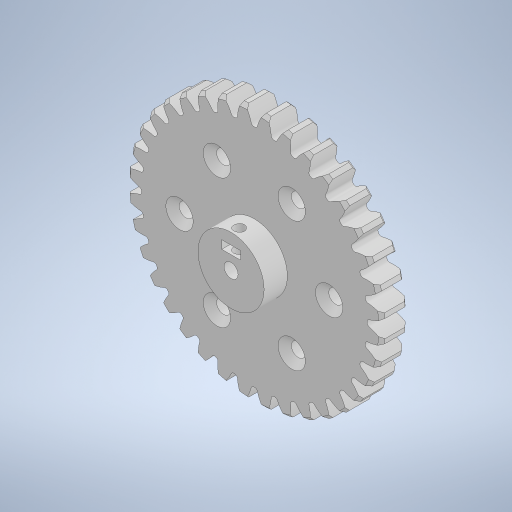
# Autodesk Inventor part: шестерня36_туу
Saved by Autodesk Inventor 2023.1 (Build 271208000, 208)
## iProperties
Created: 2025-10-14
Part Number: шестерня36_туу
Material: Generic
Document SubType Name: Modeling
Designer: DELL
Density: 1 g/cm^3
Appearance: Default
Author: DELL
Autodesk Inventor part; units mm, degrees
ref_plane "YZ Plane" through (0, 0, 0) normal (1, 0, 0) x (0, 1, 0)
ref_plane "XZ Plane" through (0, 0, 0) normal (0, 1, 0) x (-1, 0, 0)
ref_plane "XY Plane" through (0, 0, 0) normal (0, 0, 1) x (1, 0, 0)
sketch "Sketch1" plane through (0, 0, 0) normal (0, 0, 1) x (1, 0, 0)
  spline S0 degree 3 poles (-2.6391, 38.3092) (-2.5215, 38.118) (-2.2861, 37.7357) (-1.9626, 37.1448) (-1.7132, 36.642) (-1.5287, 36.2327) (-1.3982, 35.9223) (-1.2763, 35.6084) (-1.1644, 35.2908) (-1.0607, 34.9703) (-0.9922, 34.6983) (-0.9285, 34.4827) (-0.8569, 34.3297) (-0.7773, 34.2133) (-0.7005, 34.1313) (-0.6372, 34.0756) (-0.5678, 34.0277) (-0.4947, 33.9858) (-0.4163, 33.9545) (-0.3356, 33.9305) (-0.2526, 33.9149) (-0.1402, 33.9106) (0, 33.9133) (0.1402, 33.9106) (0.2526, 33.9149) (0.3356, 33.9305) (0.4163, 33.9545) (0.4947, 33.9858) (0.5678, 34.0277) (0.6372, 34.0756) (0.7005, 34.1313) (0.7773, 34.2133) (0.8569, 34.3297) (0.9285, 34.4827) (0.9922, 34.6983) (1.0607, 34.9703) (1.1644, 35.2908) (1.2763, 35.6084) (1.3982, 35.9223) (1.5287, 36.2327) (1.7132, 36.642) (1.9626, 37.1448) (2.2861, 37.7357) (2.5215, 38.118) (2.6391, 38.3092) knots 0 0 0 0 0.067335 0.13467 0.202004 0.235674 0.269343 0.303011 0.33668 0.370348 0.404017 0.420846 0.43767 0.454483 0.462902 0.471317 0.479733 0.488149 0.496564 0.50498 0.513396 0.521811 0.538646 0.555481 0.563897 0.572313 0.580729 0.589144 0.597559 0.605976 0.614391 0.622809 0.639622 0.656446 0.673275 0.706944 0.740612 0.774281 0.80795 0.841619 0.875288 0.942622 1.009957 1.077293 1.077293 1.077293 1.077293
  circle A0 centre (0, 0) radius 33.9122 construction
  circle A1 centre (0, 0) radius 33.8289 construction
  circle A2 centre (0, 0) radius 36 construction
  circle A3 centre (0, 0) radius 38.4
  point P0 (-2.291, 37.7328)
  point P1 (-1.9666, 37.1427)
  point P2 (-1.6683, 36.5391)
  point P3 (-1.53, 36.2321)
  point P4 (-1.3996, 35.9217)
  point P5 (-1.278, 35.6078)
  point P6 (-1.1658, 35.2903)
  point P7 (-1.0643, 34.9693)
  point P8 (-0.9755, 34.6445)
  point P9 (-0.9246, 34.4841)
  point P10 (-0.8529, 34.3319)
  point P11 (-0.757, 34.1938)
  point P12 (-0.6996, 34.1323)
  point P13 (-0.6362, 34.0769)
  point P14 (-0.5672, 34.0287)
  point P15 (-0.4938, 33.9875)
  point P16 (-0.4159, 33.9557)
  point P17 (-0.3352, 33.9319)
  point P18 (-0.2524, 33.917)
  point P19 (-0.1683, 33.9122)
  point P20 (0, 33.9122)
  point P21 (0.1683, 33.9122)
  point P22 (0.2524, 33.917)
  point P23 (0.3352, 33.9319)
  point P24 (0.4159, 33.9557)
  point P25 (0.4938, 33.9875)
  point P26 (0.5672, 34.0287)
  point P27 (0.6362, 34.0769)
  point P28 (0.6996, 34.1323)
  point P29 (0.757, 34.1938)
  point P30 (0.8529, 34.3319)
  point P31 (0.9246, 34.4841)
  point P32 (0.9755, 34.6445)
  point P33 (1.0643, 34.9693)
  point P34 (1.1658, 35.2903)
  point P35 (1.278, 35.6078)
  point P36 (1.3996, 35.9217)
  point P37 (1.53, 36.2321)
  point P38 (1.6683, 36.5391)
  point P39 (1.9666, 37.1427)
  point P40 (2.291, 37.7328)
  constraints: 4 centre point, 2 point on circle, 91 other
extrude "Выдавливание1" add sketch "Sketch1" against normal blind 8
extrude "Выдавливание2" cut sketch "Sketch1" against normal blind 10 contours A3 S0 picked at (-0.1561, 36.7485)
chamfer "Фаска1" distance 1 angle 45 2 edges at (0, -38.4, 0) (0, -38.4, -8)
pattern_circular "Круговой массив1" count 36 over 360 about axis through (0, 0, 0) along (0, 0, -1) of "Выдавливание2"
sketch "Эскиз2" plane through (0, 0, 0) normal (0, 0, 1) x (1, 0, 0)
  circle A0 centre (0, 0) radius 9.925
  dimension "d10" = 19.85
  constraints: 1 centre point, 1 coincident
  measures "d10" diameter of A0
extrude "Выдавливание3" add sketch "Эскиз2" along normal blind 7
sketch "Эскиз3" plane through (0, 0, 7) normal (0, 0, 1) x (1, 0, 0)
  circle A0 centre (0, 0) radius 2.1
  dimension "d13" = 4.2
  constraints: 1 centre point, 1 coincident
  measures "d13" diameter of A0
extrude "Выдавливание4" cut sketch "Эскиз3" against normal blind 20
sketch "Эскиз4" plane through (0, 0, 7) normal (0, 0, 1) x (1, 0, 0)
  line L0 (2.8, 6.6) -> (-2.8, 6.6)
  line L1 (-2.8, 6.6) -> (-2.8, 4.1)
  line L2 (-2.8, 4.1) -> (2.8, 4.1)
  line L3 (2.8, 4.1) -> (2.8, 6.6)
  line L4 (2.8, 6.6) -> (-2.8, 4.1) construction
  line L5 (-2.8, 6.6) -> (2.8, 4.1) construction
  circle A0 centre (0, 0) radius 2.1 projected
  point P0 (0, 5.35)
  dimension "d16" = 5.6
  dimension "d17" = 2.5
  dimension "d18" = 4.1
  constraints: 12 end point, 2 midpoint, 2 parallel, 1 horizontal, 1 perpendicular
  measures "d16" distance of L2.end L1.end
  measures "d17" distance of L1.end L0.end
  measures "d18" distance from line of A0.centre L2
extrude "Выдавливание5" cut sketch "Эскиз4" against normal blind 6 contours L3 L2 L1 L0
sketch "Эскиз5" plane through (-2.8, 6.6, 7) normal (0, -1, 0) x (1, 0, 0)
  circle A0 centre (2.8, -2.4) radius 1.6
  line L0 (12.725, 0) -> (-7.125, 0) projected
  point P0 (2.8, -7)
  dimension "d21" = 3.2
  dimension "d22" = 2.4
  constraints: 1 centre point
  measures "d21" diameter of A0
  measures "d22" distance from line of L0 A0.centre
extrude "Выдавливание6" cut sketch "Эскиз5" along normal mid plane 10
sketch "Эскиз6" plane through (0, 0, -8) normal (0, 0, -1) x (-1, 0, 0)
  circle A0 centre (0, 0) radius 2.1 construction
  circle A1 centre (0, 0) radius 22.5 construction
  circle A2 centre (22.5, 0) radius 2.1
  dimension "d25" = 45
  dimension "d26" = 4.2
  constraints: 1 centre point, 1 coincident, 1 horizontal alignment, 2 other
  measures "d26" diameter of A2
extrude "Выдавливание7" cut sketch "Эскиз6" against normal blind 8
pattern_circular "Круговой массив3" count 6 over 360 about axis through (0, 0, 7) along (0, 0, -1) of "Выдавливание7"
chamfer "Фаска2" distance 2 angle 45 6 edges at (-10.2, 17.6669, 0) (10.2, 17.6669, 0) (20.4, 0, 0) (10.2, -17.6669, 0) (-10.2, -17.6669, 0) (-20.4, 0, 0)
equation "\"Модуль\" = 2"
equation "\"Угол_зацепления\" = 20deg"
equation "\"Зазор_профиля_зуба\" = 0.25"
equation "\"Радиус_закругления_зуба\" = 0.35"
equation "\"Диаметр_головки\" = 76.8"
equation "\"Диаметр_впадин\" = 67.82446"
equation "\"Основной_диаметр\" = 67.65787"
equation "\"Средний_диаметр\" = 72"
equation "\"Коэффициент_смещения\" = 0.206115"
equation "\"Изменение_высоты_головки_зуба\" = 0.006115"
equation "\"Окружной_шаг\" = 6.283185"
equation "\"Общий_сдвиг_инструмента\" = 0.41223"
equation "\"Внутренний\" = 0"
